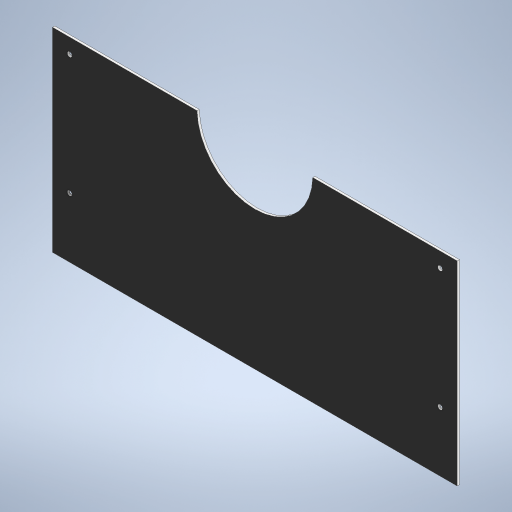
# Autodesk Inventor part: plate_top_03
Saved by Autodesk Inventor 2023 (Build 270158000, 158)
## iProperties
Created: 2023-08-22
Part Number: plate_top_03
Material: Polystyrene
Document SubType Name: Modeling
Designer: chriboehm
Density: 1.021 g/cm^3
Appearance: White
Author: chriboehm
Autodesk Inventor part; units mm, degrees
ref_plane "YZ Plane" through (0, 0, 0) normal (1, 0, 0) x (0, 1, 0)
ref_plane "XZ Plane" through (0, 0, 0) normal (0, 1, 0) x (-1, 0, 0)
ref_plane "XY Plane" through (0, 0, 0) normal (0, 0, 1) x (1, 0, 0)
sketch "Sketch1" plane through (0, 0, 0) normal (0, 0, 1) x (1, 0, 0)
  line L0 (0, 0) -> (542, 0)
  line L1 (542, 0) -> (542, 261)
  line L2 (0, 261) -> (0, 0)
  line L3 (271, 0) -> (271, 263)
  arc A0 (193.5258, 261) -> (348.4742, 261) centre (271, 263) ccw
  line L4 (542, 261) -> (348.4742, 261)
  line L5 (193.5258, 261) -> (0, 261)
  dimension "d0" = 542
  dimension "d24" = 155
  dimension "d25" = 263
  dimension "d26" = 261
  constraints: 12 end point, 3 parallel, 2 point on circle, 1 centre point, 1 coincident, 1 collinear, 1 horizontal, 1 midpoint, 1 perpendicular, 1 vertical
  measures "d0" distance of L1.end L2.start
  measures "d24" diameter of A0
  measures "d25" distance from line of L0 L3.end
  measures "d26" distance between parallel lines of L0 L5
extrude "Extrusion1" add sketch "Sketch1" along normal blind 3
sketch "Sketch2" plane through (0, 0, 0) normal (0, 0, -1) x (-1, 0, 0)
  line L0 (0, 261) -> (0, 0) projected
  line L1 (-542, 0) -> (-542, 261) projected
  line L2 (-542, 261) -> (0, 261) projected
  point P0 (-23, 241)
  point P1 (-23, 80)
  point P2 (-519, 241)
  point P3 (-519, 80)
  dimension "d4" = 23
  dimension "d13" = 20
  dimension "d14" = 261
  dimension "d15" = 542
  dimension "d18" = 161
  dimension "d21" = 496
  constraints: 1 horizontal, 1 vertical, 3 other
  measures "d4" distance from line of L0 point (-23, 241)
  measures "d13" distance from line of L2 point (-23, 241)
  measures "d14" distance of L0.start L0.end
  measures "d15" distance of L1.end L0.start
  measures "d18" distance of point (-23, 241) point (-23, 80)
  measures "d21" distance of point (-23, 241) point (-519, 241)
hole "Hole1" at (23, 241, 0) at (519, 241, 0) at (519, 80, 0) at (23, 80, 0) direction (0, 0, 1) diameter 6.5 end through all
body "Solid1"
